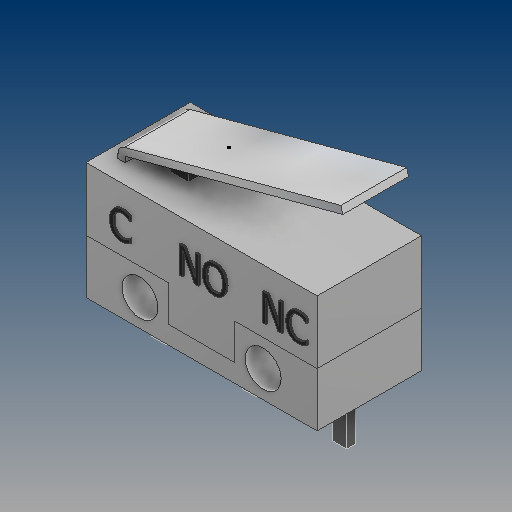
# Autodesk Inventor part: krancowka
Saved by Autodesk Inventor 2021 (Build 250183000, 183)
## iProperties
Created: 2022-05-17
Part Number: krancowka
Material: Generic
Document SubType Name: Modeling
Designer: agnpi
Density: 1 g/cm^3
Appearance: Default
Author: agnpi
Autodesk Inventor part; units mm, degrees
ref_plane "YZ Plane" through (0, 0, 0) normal (1, 0, 0) x (0, 1, 0)
ref_plane "XZ Plane" through (0, 0, 0) normal (0, 1, 0) x (-1, 0, 0)
ref_plane "XY Plane" through (0, 0, 0) normal (0, 0, 1) x (1, 0, 0)
sketch "Sketch1" plane through (0, 0, 0) normal (0, 0, 1) x (1, 0, 0)
  line L0 (-8.995, 0) -> (8.995, 0) projected
  line L1 (0, -4.9091) -> (0, 6.7045) projected
  line L2 (-6.425, 3.25) -> (6.425, 3.25)
  line L3 (6.425, 3.25) -> (6.425, -3.25)
  line L4 (6.425, -3.25) -> (-6.425, -3.25)
  line L5 (-6.425, -3.25) -> (-6.425, 3.25)
  line L6 (-6.425, 3.25) -> (6.425, -3.25) construction
  line L7 (6.425, 3.25) -> (-6.425, -3.25) construction
  point P0 (0, 0)
  dimension "d0" = 12.85
  dimension "d1" = 6.5
  constraints: 12 end point, 2 midpoint, 2 parallel, 1 horizontal, 1 perpendicular
  measures "d0" distance of L3.end L4.end
  measures "d1" distance of L2.end L3.end
extrude "Extrusion1" add sketch "Sketch1" along normal mid plane 5.8
sketch "Sketch2" plane through (0, 0, 2.9) normal (0, 0, 1) x (1, 0, 0)
  line L0 (6.425, 3.25) -> (-6.425, 3.25) projected
  line L1 (-6.425, -3.25) -> (6.425, -3.25) projected
  line L2 (-6.425, 3.25) -> (-6.425, -3.25)
  line L3 (-6.425, -3.25) -> (6.425, -3.25)
  line L4 (6.425, -3.25) -> (6.425, 3.25) projected
  line L5 (6.425, -3.25) -> (6.425, 3.25)
  line L6 (-6.425, 3.25) -> (-6.425, -3.25) projected
  line L7 (-6.425, -0.25) -> (-1.85, -0.25)
  line L8 (-1.85, -0.25) -> (-1.85, -2.25)
  line L9 (-1.85, -2.25) -> (1.85, -2.25)
  line L10 (1.85, -2.25) -> (1.85, -0.25)
  line L11 (1.85, -0.25) -> (6.425, -0.25)
  point P0 (0, 0)
  dimension "d4" = 3
  dimension "d5" = 3.7
  dimension "d6" = 2
  dimension "d7" = 4.575
  constraints: 16 end point, 4 point on line, 3 perpendicular, 2 collinear, 1 horizontal, 1 vertical
  measures "d4" distance between parallel lines of L1 L7
  measures "d5" distance between parallel lines of L10 L8
  measures "d6" distance between parallel lines of L11 L9
  measures "d7" distance between parallel lines of L2 L8
split_face "Split1"
sketch "Sketch3" plane through (-6.425, -3.25, 2.9) normal (0, 0, 1) x (1, 0, 0)
  circle A0 centre (3, 1.5) radius 1
  circle A1 centre (9.85, 1.5) radius 1
  line L0 (0, 3) -> (0, 0) projected
  line L1 (12.85, 0) -> (12.85, 3) projected
  line L2 (0, 0) -> (12.85, 0) projected
  point P0 (6.425, 3.25)
  dimension "d8" = 2
  dimension "d9" = 2
  dimension "d10" = 3
  dimension "d11" = 3
  dimension "d53" = 6.85
  dimension "d54" = 1.5
  constraints: 2 centre point
  measures "d8" diameter of A0
  measures "d9" diameter of A1
  measures "d10" distance from line of L0 A0.centre
  measures "d11" distance from line of L1 A1.centre
  measures "d53" distance of A1.centre A0.centre
  measures "d54" distance from line of L2 A0.centre
extrude "Extrusion2" cut sketch "Sketch3" against normal through all
sketch "Sketch6" plane through (0, 0, 0) normal (0, 0, 1) x (1, 0, 0)
  line L0 (-5.425, -3.25) -> (-4.625, -3.25)
  line L1 (-4.625, -3.25) -> (-4.625, -5.95)
  line L2 (-4.625, -5.95) -> (-5.425, -5.95)
  line L3 (-5.425, -5.95) -> (-5.425, -3.25)
  line L4 (-6.425, -0.25) -> (-6.425, -3.25) projected
  line L5 (-0.4, -3.25) -> (0.4, -3.25)
  line L6 (0.4, -3.25) -> (0.4, -5.95)
  line L7 (0.4, -5.95) -> (-0.4, -5.95)
  line L8 (-0.4, -5.95) -> (-0.4, -3.25)
  line L9 (4.625, -3.25) -> (5.425, -3.25)
  line L10 (5.425, -3.25) -> (5.425, -5.95)
  line L11 (5.425, -5.95) -> (4.625, -5.95)
  line L12 (4.625, -5.95) -> (4.625, -3.25)
  line L13 (-6.425, -3.25) -> (6.425, -3.25) projected
  line L14 (6.425, -3.25) -> (6.425, -0.25) projected
  point P0 (0, 0)
  dimension "d17" = 0.8
  dimension "d18" = 2.7
  dimension "d19" = 1
  dimension "d20" = 0.8
  dimension "d21" = 2.7
  dimension "d22" = 0.8
  dimension "d23" = 2.7
  dimension "d24" = 1
  dimension "d25" = 4.225
  constraints: 24 end point, 6 parallel, 3 horizontal, 3 perpendicular, 3 point on line
  measures "d17" distance between parallel lines of L1 L3
  measures "d18" distance between parallel lines of L2 L0
  measures "d19" distance between parallel lines of L3 L4
  measures "d20" distance of L6.end L7.end
  measures "d21" distance of L5.end L6.end
  measures "d22" distance of L10.end L11.end
  measures "d23" distance of L9.end L10.end
  measures "d24" distance between parallel lines of L14 L10
  measures "d25" distance between parallel lines of L8 L1
extrude "Extrusion3" add sketch "Sketch6" along normal mid plane 0.5 separate body
sketch "Sketch7" plane through (-6.425, 3.25, 2.9) normal (0, 0, 1) x (1, 0, 0)
  line L0 (5.1268, -1.1962) -> (7.9639, -1.1962) construction
  line L1 (7.9639, -1.1962) -> (7.9639, -2.7594) construction
  line L2 (7.9639, -2.7594) -> (5.1268, -2.7594) construction
  line L3 (5.1268, -2.7594) -> (5.1268, -1.1962) construction
  line L4 (1.3385, -1.1749) -> (2.5771, -1.1749) construction
  line L5 (2.5771, -1.1749) -> (2.5771, -2.7284) construction
  line L6 (2.5771, -2.7284) -> (1.3385, -2.7284) construction
  line L7 (1.3385, -2.7284) -> (1.3385, -1.1749) construction
  line L8 (9.7664, -1.1749) -> (12.3823, -1.1749) construction
  line L9 (12.3823, -1.1749) -> (12.3823, -2.7284) construction
  line L10 (12.3823, -2.7284) -> (9.7664, -2.7284) construction
  line L11 (9.7664, -2.7284) -> (9.7664, -1.1749) construction
  spline S0 degree 2 poles (2.0763, -2.7284) (1.9304, -2.7284) (1.6837, -2.63) (1.5937, -2.5315) knots 0 0 0 1 2 2 2
  spline S1 degree 2 poles (1.5937, -2.5315) (1.5038, -2.4343) (1.4053, -2.1425) (1.4053, -1.9529) knots 0 0 0 1 2 2 2
  spline S2 degree 2 poles (1.4053, -1.9529) (1.4053, -1.7645) (1.5013, -1.4849) (1.5925, -1.3816) knots 0 0 0 1 2 2 2
  spline S3 degree 2 poles (1.5925, -1.3816) (1.6825, -1.2807) (1.928, -1.1749) (2.0799, -1.1749) knots 0 0 0 1 2 2 2
  spline S4 degree 2 poles (2.0799, -1.1749) (2.1553, -1.1749) (2.2878, -1.1968) (2.3437, -1.2138) knots 0 0 0 1 2 2 2
  spline S5 degree 2 poles (2.3437, -1.2138) (2.3923, -1.2296) (2.4932, -1.2746) (2.5431, -1.3014) knots 0 0 0 1 2 2 2
  line L12 (2.5431, -1.3014) -> (2.5431, -1.542)
  line L13 (2.5431, -1.542) -> (2.5273, -1.542)
  spline S6 degree 2 poles (2.5273, -1.542) (2.5005, -1.5177) (2.4179, -1.4497) (2.3583, -1.4168) knots 0 0 0 1 2 2 2
  spline S7 degree 2 poles (2.3583, -1.4168) (2.3012, -1.3852) (2.1662, -1.3451) (2.0787, -1.3451) knots 0 0 0 1 2 2 2
  spline S8 degree 2 poles (2.0787, -1.3451) (1.9827, -1.3451) (1.8113, -1.4241) (1.7469, -1.4995) knots 0 0 0 1 2 2 2
  spline S9 degree 2 poles (1.7469, -1.4995) (1.6837, -1.5761) (1.6132, -1.8082) (1.6132, -1.9529) knots 0 0 0 1 2 2 2
  spline S10 degree 2 poles (1.6132, -1.9529) (1.6132, -2.1073) (1.6873, -2.3297) (1.7517, -2.4063) knots 0 0 0 1 2 2 2
  spline S11 degree 2 poles (1.7517, -2.4063) (1.815, -2.4805) (1.9839, -2.5558) (2.0787, -2.5558) knots 0 0 0 1 2 2 2
  spline S12 degree 2 poles (2.0787, -2.5558) (2.165, -2.5558) (2.3121, -2.5133) (2.3692, -2.4817) knots 0 0 0 1 2 2 2
  spline S13 degree 2 poles (2.3692, -2.4817) (2.4239, -2.4501) (2.5054, -2.3844) (2.5285, -2.3613) knots 0 0 0 1 2 2 2
  line L14 (2.5285, -2.3613) -> (2.5431, -2.3613)
  line L15 (2.5431, -2.3613) -> (2.5431, -2.5996)
  spline S14 degree 2 poles (2.5431, -2.5996) (2.4932, -2.6227) (2.4057, -2.6652) (2.3437, -2.6847) knots 0 0 0 1 2 2 2
  spline S15 degree 2 poles (2.3437, -2.6847) (2.2781, -2.7065) (2.1662, -2.7284) (2.0763, -2.7284) knots 0 0 0 1 2 2 2
  line L16 (6.352, -2.7278) -> (6.1284, -2.7278)
  line L17 (6.1284, -2.7278) -> (5.4647, -1.4345)
  line L18 (5.4647, -1.4345) -> (5.4647, -2.7278)
  line L19 (5.4647, -2.7278) -> (5.2787, -2.7278)
  line L20 (5.2787, -2.7278) -> (5.2787, -1.2278)
  line L21 (5.2787, -1.2278) -> (5.5619, -1.2278)
  line L22 (5.5619, -1.2278) -> (6.1661, -2.4154)
  line L23 (6.1661, -2.4154) -> (6.1661, -1.2278)
  line L24 (6.1661, -1.2278) -> (6.352, -1.2278)
  line L25 (6.352, -1.2278) -> (6.352, -2.7278)
  spline S16 degree 2 poles (7.7171, -1.3992) (7.8022, -1.4989) (7.897, -1.7906) (7.897, -1.9778) knots 0 0 0 1 2 2 2
  spline S17 degree 2 poles (7.897, -1.9778) (7.897, -2.1602) (7.8046, -2.4555) (7.7171, -2.5552) knots 0 0 0 1 2 2 2
  spline S18 degree 2 poles (7.7171, -2.5552) (7.6247, -2.6598) (7.3804, -2.7594) (7.2333, -2.7594) knots 0 0 0 1 2 2 2
  spline S19 degree 2 poles (7.2333, -2.7594) (7.0814, -2.7594) (6.8383, -2.6561) (6.7495, -2.5552) knots 0 0 0 1 2 2 2
  spline S20 degree 2 poles (6.7495, -2.5552) (6.6632, -2.4555) (6.5708, -2.1626) (6.5708, -1.9778) knots 0 0 0 1 2 2 2
  spline S21 degree 2 poles (6.5708, -1.9778) (6.5708, -1.7894) (6.6644, -1.5025) (6.7507, -1.3992) knots 0 0 0 1 2 2 2
  spline S22 degree 2 poles (6.7507, -1.3992) (6.8383, -1.2995) (7.0826, -1.1962) (7.2333, -1.1962) knots 0 0 0 1 2 2 2
  spline S23 degree 2 poles (7.2333, -1.1962) (7.3865, -1.1962) (7.632, -1.3032) (7.7171, -1.3992) knots 0 0 0 1 2 2 2
  spline S24 degree 2 poles (7.6892, -1.9778) (7.6892, -1.8295) (7.6247, -1.5998) (7.5664, -1.5244) knots 0 0 0 1 2 2 2
  spline S25 degree 2 poles (7.5664, -1.5244) (7.5068, -1.4466) (7.3391, -1.3688) (7.2345, -1.3688) knots 0 0 0 1 2 2 2
  spline S26 degree 2 poles (7.2345, -1.3688) (7.1264, -1.3688) (6.9635, -1.4442) (6.9015, -1.5244) knots 0 0 0 1 2 2 2
  spline S27 degree 2 poles (6.9015, -1.5244) (6.8419, -1.601) (6.7787, -1.832) (6.7787, -1.9778) knots 0 0 0 1 2 2 2
  spline S28 degree 2 poles (6.7787, -1.9778) (6.7787, -2.2732) (7.0267, -2.5868) (7.2345, -2.5868) knots 0 0 0 1 2 2 2
  spline S29 degree 2 poles (7.2345, -2.5868) (7.4424, -2.5868) (7.6892, -2.2732) (7.6892, -1.9778) knots 0 0 0 1 2 2 2
  line L26 (10.9917, -2.7017) -> (10.768, -2.7017)
  line L27 (10.768, -2.7017) -> (10.1043, -1.4083)
  line L28 (10.1043, -1.4083) -> (10.1043, -2.7017)
  line L29 (10.1043, -2.7017) -> (9.9183, -2.7017)
  line L30 (9.9183, -2.7017) -> (9.9183, -1.2017)
  line L31 (9.9183, -1.2017) -> (10.2015, -1.2017)
  line L32 (10.2015, -1.2017) -> (10.8057, -2.3893)
  line L33 (10.8057, -2.3893) -> (10.8057, -1.2017)
  line L34 (10.8057, -1.2017) -> (10.9917, -1.2017)
  line L35 (10.9917, -1.2017) -> (10.9917, -2.7017)
  spline S30 degree 2 poles (11.8814, -2.7284) (11.7356, -2.7284) (11.4888, -2.63) (11.3989, -2.5315) knots 0 0 0 1 2 2 2
  spline S31 degree 2 poles (11.3989, -2.5315) (11.3089, -2.4343) (11.2105, -2.1425) (11.2105, -1.9529) knots 0 0 0 1 2 2 2
  spline S32 degree 2 poles (11.2105, -1.9529) (11.2105, -1.7645) (11.3065, -1.4849) (11.3977, -1.3816) knots 0 0 0 1 2 2 2
  spline S33 degree 2 poles (11.3977, -1.3816) (11.4876, -1.2807) (11.7331, -1.1749) (11.8851, -1.1749) knots 0 0 0 1 2 2 2
  spline S34 degree 2 poles (11.8851, -1.1749) (11.9605, -1.1749) (12.093, -1.1968) (12.1489, -1.2138) knots 0 0 0 1 2 2 2
  spline S35 degree 2 poles (12.1489, -1.2138) (12.1975, -1.2296) (12.2984, -1.2746) (12.3482, -1.3014) knots 0 0 0 1 2 2 2
  line L36 (12.3482, -1.3014) -> (12.3482, -1.542)
  line L37 (12.3482, -1.542) -> (12.3324, -1.542)
  spline S36 degree 2 poles (12.3324, -1.542) (12.3057, -1.5177) (12.223, -1.4497) (12.1635, -1.4168) knots 0 0 0 1 2 2 2
  spline S37 degree 2 poles (12.1635, -1.4168) (12.1063, -1.3852) (11.9714, -1.3451) (11.8839, -1.3451) knots 0 0 0 1 2 2 2
  spline S38 degree 2 poles (11.8839, -1.3451) (11.7878, -1.3451) (11.6165, -1.4241) (11.552, -1.4995) knots 0 0 0 1 2 2 2
  spline S39 degree 2 poles (11.552, -1.4995) (11.4888, -1.5761) (11.4183, -1.8082) (11.4183, -1.9529) knots 0 0 0 1 2 2 2
  spline S40 degree 2 poles (11.4183, -1.9529) (11.4183, -2.1073) (11.4925, -2.3297) (11.5569, -2.4063) knots 0 0 0 1 2 2 2
  spline S41 degree 2 poles (11.5569, -2.4063) (11.6201, -2.4805) (11.7891, -2.5558) (11.8839, -2.5558) knots 0 0 0 1 2 2 2
  spline S42 degree 2 poles (11.8839, -2.5558) (11.9702, -2.5558) (12.1173, -2.5133) (12.1744, -2.4817) knots 0 0 0 1 2 2 2
  spline S43 degree 2 poles (12.1744, -2.4817) (12.2291, -2.4501) (12.3105, -2.3844) (12.3336, -2.3613) knots 0 0 0 1 2 2 2
  line L38 (12.3336, -2.3613) -> (12.3482, -2.3613)
  line L39 (12.3482, -2.3613) -> (12.3482, -2.5996)
  spline S44 degree 2 poles (12.3482, -2.5996) (12.2984, -2.6227) (12.2109, -2.6652) (12.1489, -2.6847) knots 0 0 0 1 2 2 2
  spline S45 degree 2 poles (12.1489, -2.6847) (12.0832, -2.7065) (11.9714, -2.7284) (11.8814, -2.7284) knots 0 0 0 1 2 2 2
  point P0 (6.425, -3.25)
  constraints: 6 other
extrude "Extrusion4" add sketch "Sketch7" along normal blind 0.1 separate body
sketch "Sketch8" plane through (-6.425, 3.25, 2.9) normal (0, 1, 0) x (1, 0, 0)
  line L0 (2.8, 3.9) -> (3.8, 3.9)
  line L1 (3.8, 3.9) -> (3.8, 1.9)
  line L2 (3.8, 1.9) -> (2.8, 1.9)
  line L3 (2.8, 1.9) -> (2.8, 3.9)
  line L4 (0, 5.8) -> (0, 0) projected
  line L5 (0, 5.8) -> (12.85, 5.8) projected
  point P0 (6.425, 2.9)
  dimension "d30" = 1
  dimension "d31" = 2
  dimension "d32" = 2.8
  dimension "d33" = 1.9
  constraints: 8 end point, 2 parallel, 1 horizontal, 1 perpendicular
  measures "d30" distance of L1.end L2.end
  measures "d31" distance of L0.end L1.end
  measures "d32" distance between parallel lines of L4 L3
  measures "d33" distance between parallel lines of L5 L0
extrude "Extrusion5" add sketch "Sketch8" along normal blind 1 separate body
fillet "Fillet1" radius 0.5 2 edges at (-3.625, 4.25, 0) (-2.625, 4.25, 0)
sketch "Sketch9" plane through (-6.425, 3.25, 2.9) normal (0, 1, 0) x (1, 0, 0)
  line L0 (0.7, 4.725) -> (1.1, 4.725)
  line L1 (1.1, 4.725) -> (1.1, 1.075)
  line L2 (1.1, 1.075) -> (0.7, 1.075)
  line L3 (0.7, 1.075) -> (0.7, 4.725)
  line L4 (0, 5.8) -> (12.85, 5.8) projected
  line L5 (0, 5.8) -> (0, 0) projected
  point P0 (6.425, 2.9)
  dimension "d37" = 0.4
  dimension "d38" = 3.65
  dimension "d39" = 1.075
  dimension "d40" = 0.7
  constraints: 8 end point, 2 parallel, 1 horizontal, 1 perpendicular
  measures "d37" distance between parallel lines of L1 L3
  measures "d38" distance between parallel lines of L2 L0
  measures "d39" distance between parallel lines of L4 L0
  measures "d40" distance between parallel lines of L5 L3
sketch "Sketch10" plane through (0, 0, 0) normal (0, 0, 1) x (1, 0, 0)
  line L0 (-5.525, 3.25) -> (-5.525, 3.5)
  line L1 (-6.425, -0.25) -> (-6.425, 3.25) projected
  line L2 (-6.425, 3.25) -> (6.425, 3.25)
  arc A0 (-5.3116, 3.7774) -> (-5.525, 3.5) centre (-5.238, 3.5) ccw
  line L3 (-5.3116, 3.7774) -> (6.725, 7.0026)
  point P0 (0, 0)
  dimension "d41" = 0.25
  dimension "d42" = 0.9
  dimension "d45" = 0.287
  dimension "d46" = 0.25
  dimension "d47" = 0.287
  dimension "d48" = 0.35
  dimension "d49" = 12.25
  dimension "d50" = 15
  constraints: 6 end point, 2 point on circle, 1 centre point, 1 vertical
  measures "d41" distance of L0.start L0.end
  measures "d42" distance from line of L1.end L0
  measures "d45" radius of A0
  measures "d46" distance from line of L2 A0.centre
  measures "d47" distance from line of L0 A0.centre
  measures "d48" distance of L3.start L0.end
  measures "d49" distance from line of L3.end L0
  measures "d50" angle of L2 L3
sweep "Sweep1" add profiles "Sketch9" path "Sketch10" bodies 1 path curves L0 A0 L3
sketch "Sketch11" plane through (-5.3629, 3.9707, 1.825) normal (-0.2588, 0.9659, 0) x (0.9659, 0.2588, 0)
  point P0 (4.1524, 1.825)
body "Solid1"
body "Solid2"
body "Solid3"
body "Solid4"
